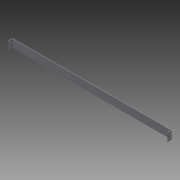
# Autodesk Inventor part: bumper piece
Saved by Autodesk Inventor 2015 (Build 190159000, 159)
## iProperties
Created: 2015-01-31
Part Number: bumper piece
Material: Generic
Document SubType Name: Sheet Metal
Designer: mastkee16
Density: 1 g/cm^3
Flat Pattern Width: 5.08 cm
Flat Pattern Length: 106.813 cm
Flat Pattern Area: 542.61 cm^2
Sheet Metal Rule: Default
Sheet Metal Width: 2.000 in
Sheet Metal Length: 42.052 in
Sheet Metal Area: 84.105 in^2
Appearance: Default
Author: mastkee16
Autodesk Inventor part; units mm, degrees
ref_plane "YZ Plane" through (0, 0, 0) normal (1, 0, 0) x (0, 1, 0)
ref_plane "XZ Plane" through (0, 0, 0) normal (0, 1, 0) x (-1, 0, 0)
ref_plane "XY Plane" through (0, 0, 0) normal (0, 0, 1) x (1, 0, 0)
sketch "Sketch1" plane through (0, 0, 0) normal (0, 0, 1) x (1, 0, 0)
  line L0 (0, 0) -> (1021.08, 0)
  line L1 (1021.08, 0) -> (1021.08, 50.8)
  line L2 (1021.08, 50.8) -> (0, 50.8)
  line L3 (0, 50.8) -> (0, 0)
  dimension "d0" = 1021.08
  dimension "d1" = 50.8
  measures "d0" distance of L2.end L1.end
  measures "d1" distance of L1.end L0.end
extrude "Plate1" add sketch "Sketch1" along normal blind 2.54
sketch "Sketch2" plane through (2.54, 0, 0) normal (-1, 0, 0) x (0, -1, 0)
  line L0 (-50.8, 0) -> (0, 0)
  line L1 (0, 0) -> (0, 27.94)
  line L2 (0, 27.94) -> (-50.8, 27.94)
  line L3 (-50.8, 27.94) -> (-50.8, 0)
  constraints: 6 end point, 1 horizontal, 1 perpendicular, 1 vertical
edge flange "Flange1" height 27.94 angle 90 thickness 2.54 bend radius 2.54 thickness toward (-1, 0, 0) relief tear relief width 2.54 relief depth 1.27 corner gap 2.54 corner form 0 edges at (0, 25.4, 2.54) (1021.08, 25.4, 2.54) wall of the first edge with corners at (2.54, 50.8, 0) (2.54, 0, 0) (2.54, 0, 27.94) (2.54, 50.8, 27.94)
bend "Bend1"
corner "Corner1"
sketch "Sketch3" plane through (0, 0, 0) normal (0, 0, -1) x (-1, 0, 0)
  circle A0 centre (-317.326, 37.1303) radius 3.175 projected
  circle A1 centre (-657.3374, 25.4) radius 3.175 projected
  circle A2 centre (-363.7426, 25.4) radius 3.175 projected
  point P0 (0, 0)
extrude "Extrusion1" cut sketch "Sketch3" against normal blind 25.4 contours A1 | A2
sketch "Sketch4" plane through (1021.08, 0, 27.94) normal (1, 0, 0) x (0, 0, -1)
  line L0 (0, 0) -> (22.86, 0)
  line L1 (22.86, 0) -> (22.86, 50.8)
  line L2 (22.86, 50.8) -> (0, 50.8)
  line L3 (0, 50.8) -> (0, 0)
  circle A0 centre (11.43, 38.1) radius 3.175
  circle A1 centre (11.43, 12.7) radius 3.175
  point P0 (27.94, 0)
  dimension "d15" = 6.35
  dimension "d16" = 6.35
  constraints: 8 end point, 2 centre point, 2 coincident, 2 parallel, 1 horizontal, 1 perpendicular
  measures "d15" diameter of A0
  measures "d16" diameter of A1
extrude "Extrusion2" cut sketch "Sketch4" against normal blind 2.54 contours A0 | A1
sketch "Sketch5" plane through (0, 0, 27.94) normal (-1, 0, 0) x (0, 0, 1)
  line L0 (0, 50.8) -> (-22.86, 50.8)
  line L1 (-22.86, 50.8) -> (-22.86, 0)
  line L2 (-22.86, 0) -> (0, 0)
  line L3 (0, 0) -> (0, 50.8)
  circle A0 centre (-11.43, 38.1) radius 3.175 projected
  circle A1 centre (-11.43, 12.7) radius 3.175 projected
  circle A2 centre (-11.43, 12.7) radius 3.175
  circle A3 centre (-11.43, 38.1) radius 3.175
  point P0 (-27.94, 0)
  constraints: 8 end point, 3 coincident, 2 centre point, 2 parallel, 1 concentric, 1 horizontal, 1 perpendicular
extrude "Extrusion3" cut sketch "Sketch5" against normal blind 2.54 contours A0 | A1
equation "\"d3\" = BendReliefWidth"
equation "\"d4\" = BendReliefDepth"
equation "\"d5\" = MinimumRemnant"
equation "\"d6\" = BendRadius"
equation "\"d9\" = BendRadius"
equation "\"d10\" = CornerReliefSize"
equation "\"d11\" = GapSize"
equation "\"d12\" = JacobiRadiusSize"
equation "\"BendRadius\" = Thickness"
equation "\"BendReliefWidth\" = Thickness"
equation "\"BendReliefDepth\" = 0.5 * Thickness"
equation "\"CornerReliefSize\" = 4 * Thickness"
equation "\"MinimumRemnant\" = 2 * Thickness"
equation "\"TransitionRadius\" = BendRadius"
equation "\"JacobiRadiusSize\" = BendRadius"
equation "\"GapSize\" = Thickness"
equation "\"d2\" = BendRadius"
equation "\"Thickness\" = 2.54"
body "Solid1"
